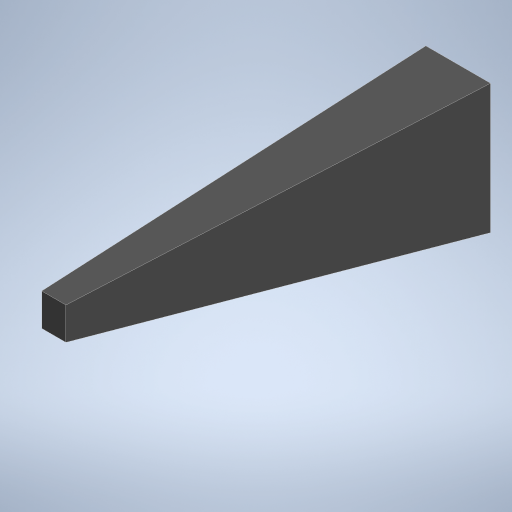
# Autodesk Inventor part: amtana
Saved by Autodesk Inventor 2024.1 (Build 281209000, 209)
## iProperties
Created: 2024-02-25
Part Number: amtana
Material: 一般
Document SubType Name: Modeling
Designer: hibik
Density: 1 g/cm^3
Appearance: 既定
Author: hibik
Autodesk Inventor part; units mm, degrees
ref_plane "YZ Plane" through (0, 0, 0) normal (1, 0, 0) x (0, 1, 0)
ref_plane "XZ Plane" through (0, 0, 0) normal (0, 1, 0) x (-1, 0, 0)
ref_plane "XY Plane" through (0, 0, 0) normal (0, 0, 1) x (1, 0, 0)
sketch "スケッチ1" plane through (0, 0, 0) normal (0, 0, 1) x (1, 0, 0)
  line L0 (-2, 8) -> (2, 8)
  line L1 (2, 8) -> (2, 0)
  line L2 (2, 0) -> (-2, 0)
  line L3 (-2, 0) -> (-2, 8)
  point P0 (0, 0)
  point P1 (0, 0)
  dimension "d0" = 8
  dimension "d1" = 4
  constraints: 8 end point, 2 parallel, 1 coincident, 1 horizontal, 1 midpoint, 1 perpendicular
  measures "d0" distance of L2.end L0.start
  measures "d1" distance of L0.start L0.end
extrude "押し出し1" add sketch "スケッチ1" along normal blind 25
sketch "スケッチ2" plane through (-2, 0, 0) normal (-1, 0, 0) x (0, 0, 1)
  line L0 (0, 0) -> (25, 6)
  line L1 (25, 0) -> (25, 8) projected
  line L2 (0, 8) -> (25, 8) projected
  line L3 (25, 8) -> (0, 8)
  line L4 (0, 8) -> (0, 0)
  line L5 (0, 8) -> (0, 0) projected
  line L6 (0, 0) -> (25, 0) projected
  line L7 (25, 8) -> (25, 0) projected
  line L8 (0, 8) -> (25, 8) projected
  point P0 (0, 0)
  dimension "d4" = 2
  constraints: 6 end point, 1 collinear, 1 perpendicular, 1 point on line
  measures "d4" distance from line of L2 L0.end
extrude "押し出し2" cut sketch "スケッチ2" against normal through all contours L0 L1 L6
sketch "スケッチ3" plane through (-2, 8, 0) normal (0, 1, 0) x (1, 0, 0)
  line L0 (4, 0) -> (4, -25) projected
  line L1 (4, 0) -> (2.75, -25)
  line L2 (2.75, -25) -> (1.25, -25)
  line L3 (1.25, -25) -> (0, 0)
  line L4 (4, 0) -> (0, 0) projected
  line L5 (4, -25) -> (0, -25) projected
  line L6 (4, 0) -> (0, 0) projected
  line L7 (0, 0) -> (0, -25) projected
  line L8 (4, -25) -> (0, -25) projected
  line L9 (4, 0) -> (4, -25) projected
  point P0 (2, 0)
  point P1 (2, -25)
  point P2 (2, 0)
  dimension "d7" = 1.5
  constraints: 6 end point, 2 midpoint, 1 collinear, 1 vertical alignment
  measures "d7" distance of L1.end L2.end
extrude "押し出し3" cut sketch "スケッチ3" against normal through all contours L0 L5 L1 | L3 L5 L7
